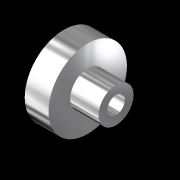
# Autodesk Inventor part: StepperAdapter
Saved by Autodesk Inventor 2018 (Build 220112000, 112)
## iProperties
Created: 2022-02-18
Part Number: StepperAdapter
Material: Aluminum 6061
Document SubType Name: Modeling
Designer: kumpu
Density: 2.7 g/cm^3
Appearance: Aluminum - Flat
Author: kumpu
Autodesk Inventor part; units mm, degrees
ref_plane "YZ Plane" through (0, 0, 0) normal (1, 0, 0) x (0, 1, 0)
ref_plane "XZ Plane" through (0, 0, 0) normal (0, 1, 0) x (-1, 0, 0)
ref_plane "XY Plane" through (0, 0, 0) normal (0, 0, 1) x (1, 0, 0)
sketch "Sketch1" plane through (0, 0, 0) normal (0, 1, 0) x (-1, 0, 0)
  line L0 (0, 0) -> (-18.923, 0)
  line L1 (0, 3.175) -> (-18.923, 3.175)
  line L2 (-18.923, 3.175) -> (-18.923, 6.35)
  line L3 (-18.923, 6.35) -> (-8.636, 6.35)
  line L4 (-8.636, 6.35) -> (-8.636, 14.224)
  line L5 (-8.636, 14.224) -> (0, 14.224)
  line L6 (0, 14.224) -> (0, 3.175)
  dimension "d0" = 12.7
  dimension "d1" = 6.35
  dimension "d2" = 10.287
  dimension "d4" = 28.448
  dimension "d5" = 8.636
  constraints: 14 end point, 5 perpendicular, 2 horizontal, 2 point on line
  measures "d0" diameter of L3 L0
  measures "d1" diameter of L1 L0
  measures "d2" distance of L2.end L3.end
  measures "d4" diameter of L5 L0
  measures "d5" distance of L4.end L5.end
revolve "Revolution1" add sketch "Sketch1" angle 360 about axis through (0, 0, 0) along (1, 0, 0)
body "Solid1"
